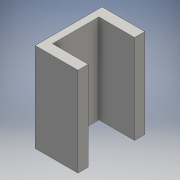
# Autodesk Inventor part: StepperDriverA4988
Saved by Autodesk Inventor 2016 (Build 200138000, 138)
## iProperties
Created: 2015-10-25
Part Number: StepperDriverA4988
Material: Generic
Document SubType Name: Modeling
Designer: Jack
Density: 1 g/cm^3
Appearance: Default
Author: Jack
Autodesk Inventor part; units mm, degrees
ref_plane "YZ Plane" through (0, 0, 0) normal (1, 0, 0) x (0, 1, 0)
ref_plane "XZ Plane" through (0, 0, 0) normal (0, 1, 0) x (-1, 0, 0)
ref_plane "XY Plane" through (0, 0, 0) normal (0, 0, 1) x (1, 0, 0)
sketch "Sketch1" plane through (0, 0, 0) normal (1, 0, 0) x (0, 1, 0)
  line L0 (0, 0) -> (15, 0)
  line L1 (15, 0) -> (15, -20)
  line L2 (15, -20) -> (0, -20)
  line L3 (0, -20) -> (0, 0)
  dimension "d0" = 15
  dimension "d1" = 20
  constraints: 8 end point, 2 parallel, 1 horizontal, 1 perpendicular
  measures "d0" distance of L1.end L2.end
  measures "d1" distance of L0.end L1.end
extrude "Extrusion1" add sketch "Sketch1" along normal blind 1.6
sketch "Sketch2" plane through (1.6, 0, 0) normal (1, 0, 0) x (0, 0, -1)
  line L0 (0, 15) -> (0, 0) projected
  line L1 (0, 0) -> (20, 0) projected
  line L2 (20, 0) -> (20, 15) projected
  line L3 (20, 15) -> (0, 15) projected
  line L4 (0, 15) -> (20, 15)
  line L5 (20, 15) -> (20, 12.7)
  line L6 (20, 12.7) -> (0, 12.7)
  line L7 (0, 12.7) -> (0, 15)
  line L8 (20, 0) -> (0, 0)
  line L9 (0, 0) -> (0, 2.3)
  line L10 (0, 2.3) -> (20, 2.3)
  line L11 (20, 2.3) -> (20, 0)
  dimension "d4" = 2.3
  dimension "d5" = 2.3
  constraints: 16 end point, 4 parallel, 2 horizontal, 2 perpendicular, 2 point on line
  measures "d4" distance between parallel lines of L3 L6
  measures "d5" distance between parallel lines of L1 L10
extrude "Extrusion2" add sketch "Sketch2" along normal blind 8 contours L3 L2 L6 L0 | L10 L2 L1 L0
equation "\"d5\" = d4"
body "Solid1"
